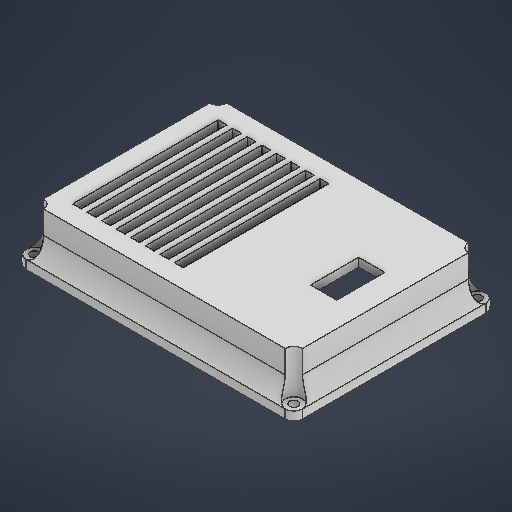
# Autodesk Inventor part: back_cover
Saved by Autodesk Inventor 2026.1 (Build 301233000, 233)
## iProperties
Created: 2026-04-26
Part Number: back_cover
Material: Generic
Document SubType Name: Modeling
Designer: emanuel
Density: 1 g/cm^3
Appearance: Default
Author: emanuel
Autodesk Inventor part; units mm, degrees
ref_plane "YZ Plane" through (0, 0, 0) normal (1, 0, 0) x (0, 1, 0)
ref_plane "XZ Plane" through (0, 0, 0) normal (0, 1, 0) x (-1, 0, 0)
ref_plane "XY Plane" through (0, 0, 0) normal (0, 0, 1) x (1, 0, 0)
sketch "Sketch1" plane through (0, 0, 0) normal (0, 1, 0) x (-1, 0, 0)
  circle A0 centre (44.5, 31.5) radius 1.5
  circle A1 centre (44.5, -31.5) radius 1.5
  circle A2 centre (-44.5, 31.5) radius 1.5
  circle A3 centre (-44.5, -31.5) radius 1.5
  line L0 (44.5, 31.5) -> (44.5, -31.5) construction
  line L1 (41.5, 31.5) -> (41.5, -31.5)
  line L2 (47.5, -31.5) -> (47.5, 31.5)
  arc A4 (47.5, 31.5) -> (41.5, 31.5) centre (44.5, 31.5) ccw
  arc A5 (41.5, -31.5) -> (47.5, -31.5) centre (44.5, -31.5) ccw
  line L3 (44.5, -31.5) -> (-44.5, -31.5) construction
  line L4 (44.5, -28.5) -> (-44.5, -28.5)
  line L5 (-44.5, -34.5) -> (44.5, -34.5)
  arc A6 (44.5, -34.5) -> (44.5, -28.5) centre (44.5, -31.5) ccw
  arc A7 (-44.5, -28.5) -> (-44.5, -34.5) centre (-44.5, -31.5) ccw
  line L6 (-44.5, -31.5) -> (-44.5, 31.5) construction
  line L7 (-41.5, -31.5) -> (-41.5, 31.5)
  line L8 (-47.5, 31.5) -> (-47.5, -31.5)
  arc A8 (-47.5, -31.5) -> (-41.5, -31.5) centre (-44.5, -31.5) ccw
  arc A9 (-41.5, 31.5) -> (-47.5, 31.5) centre (-44.5, 31.5) ccw
  line L9 (-44.5, 31.5) -> (44.5, 31.5) construction
  line L10 (-44.5, 28.5) -> (44.5, 28.5)
  line L11 (44.5, 34.5) -> (-44.5, 34.5)
  arc A10 (-44.5, 34.5) -> (-44.5, 28.5) centre (-44.5, 31.5) ccw
  arc A11 (44.5, 28.5) -> (44.5, 34.5) centre (44.5, 31.5) ccw
  point P0 (44.5, 0)
  point P1 (0, -31.5)
  point P2 (-44.5, 0)
  point P3 (0, 31.5)
  point P4 (41.5, -28.5)
  point P5 (-41.5, -28.5)
  point P6 (-41.5, 28.5)
  point P7 (41.5, 28.5)
  dimension "d2" = 3
  dimension "d3" = 3
  dimension "d4" = 3
  dimension "d5" = 3
  dimension "d6" = 6
  dimension "d7" = 6
  dimension "d8" = 6
  dimension "d9" = 6
  constraints: 32 end point, 16 point on circle, 16 tangent, 12 centre point, 4 midpoint, 4 parallel, 3 perpendicular, 1 vertical
  measures "d2" diameter of A0
  measures "d3" diameter of A1
  measures "d4" diameter of A2
  measures "d5" diameter of A3
  measures "d6" diameter of A5
  measures "d7" diameter of A7
  measures "d8" diameter of A9
  measures "d9" diameter of A11
extrude "Extrusion1" add sketch "Sketch1" along normal blind 3 contours A4 A11 L10 L1 | L1 L10 L7 A9 L11 A4 | L10 A11 L2 A6 L4 L1 | L4 A6 A5 L1 | L1 A5 L5 A8 L7 L4 | L10 A10 A9 L7 | L7 L4 A7 L8 A10 L10 | L7 A8 A7 L4
sketch "Sketch3" plane through (0, 3, 0) normal (0, 1, 0) x (1, 0, 0)
  line L0 (-41.5, -28.5) -> (-41.5, 28.5) projected
  line L1 (41.5, 28.5) -> (41.5, -28.5) projected
  line L2 (-41.5, 28.5) -> (41.5, 28.5)
  line L3 (41.5, 28.5) -> (41.5, -28.5)
  line L4 (41.5, -28.5) -> (-41.5, -28.5)
  line L5 (-41.5, -28.5) -> (-41.5, 28.5)
  circle A0 centre (-44.5, 31.5) radius 1.5 projected
  line L6 (-41.5, 28.5) -> (-44.5, 28.5)
  line L7 (-44.5, 28.5) -> (-44.5, 31.5)
  line L8 (-44.5, 31.5) -> (-41.5, 31.5)
  line L9 (-41.5, 31.5) -> (-41.5, 28.5)
  circle A1 centre (44.5, -31.5) radius 1.5 projected
  line L10 (41.5, -28.5) -> (44.5, -28.5)
  line L11 (44.5, -28.5) -> (44.5, -31.5)
  line L12 (44.5, -31.5) -> (41.5, -31.5)
  line L13 (41.5, -31.5) -> (41.5, -28.5)
  line L14 (44.5, -31.5) -> (-44.5, -31.5)
  line L15 (-44.5, -31.5) -> (-44.5, 31.5)
  line L16 (-44.5, 31.5) -> (44.5, 31.5)
  line L17 (44.5, 31.5) -> (44.5, -31.5)
  line L18 (44.5, 34.5) -> (-44.5, 34.5) projected
  circle A2 centre (-44.5, 31.5) radius 3
  circle A3 centre (-44.5, -31.5) radius 1.5 projected
  arc A4 (-47.5, -31.5) -> (-44.5, -34.5) centre (-44.5, -31.5) ccw projected
  circle A5 centre (-44.5, -31.5) radius 3
  arc A6 (44.5, -34.5) -> (47.5, -31.5) centre (44.5, -31.5) ccw projected
  circle A7 centre (44.5, -31.5) radius 3
  circle A8 centre (44.5, 31.5) radius 3
  point P0 (0, 0)
  point P1 (-44.5, -28.5)
  point P2 (-41.5, -31.5)
  point P3 (44.5, 28.5)
  point P4 (41.5, 31.5)
  constraints: 32 end point, 8 parallel, 4 coincident, 4 horizontal, 4 perpendicular, 1 centre point, 9 other
extrude "Extrusion3" add sketch "Sketch3" along normal blind 15 contours L4 L13 L14 A5 L15 L6 L0 | L9 L16 A8 L17 L10 L1 L2 | L6 A2 L9 | L10 A7 L13
fillet "Fillet2" radius 10 4 edges at (0, 3, 31.5) (44.5, 3, 0) (0, 3, -31.5) (-44.5, 3, 0)
sketch "Sketch4" plane through (0, 18, 0) normal (0, 1, 0) x (1, 0, 0)
  line L0 (41.5, 28.5) -> (41.5, -28.5) projected
  line L1 (41.5, 0) -> (31.5, 0)
  line L2 (27, -8.25) -> (36, -8.25)
  line L3 (36, -8.25) -> (36, 8.25)
  line L4 (36, 8.25) -> (27, 8.25)
  line L5 (27, 8.25) -> (27, -8.25)
  line L6 (27, -8.25) -> (36, 8.25) construction
  line L7 (36, -8.25) -> (27, 8.25) construction
  line L8 (-41.5, -28.5) -> (-41.5, 28.5) projected
  line L9 (-41.5, 0) -> (-31.5, 0)
  line L10 (-31.5, 0) -> (-21.5, 0)
  line L11 (-21.5, 0) -> (-11.5, 0)
  line L12 (-11.5, 0) -> (-1.5, 0)
  line L13 (-38, -25) -> (-35, -25)
  line L14 (-35, -25) -> (-35, 25)
  line L15 (-35, 25) -> (-38, 25)
  line L16 (-38, 25) -> (-38, -25)
  line L17 (-38, -25) -> (-35, 25) construction
  line L18 (-35, -25) -> (-38, 25) construction
  line L19 (-33, -25) -> (-30, -25)
  line L20 (-30, -25) -> (-30, 25)
  line L21 (-30, 25) -> (-33, 25)
  line L22 (-33, 25) -> (-33, -25)
  line L23 (-33, -25) -> (-30, 25) construction
  line L24 (-30, -25) -> (-33, 25) construction
  line L25 (-18, -25) -> (-15, -25)
  line L26 (-15, -25) -> (-15, 25)
  line L27 (-15, 25) -> (-18, 25)
  line L28 (-18, 25) -> (-18, -25)
  line L29 (-18, -25) -> (-15, 25) construction
  line L30 (-15, -25) -> (-18, 25) construction
  line L31 (-23, -25) -> (-20, -25)
  line L32 (-20, -25) -> (-20, 25)
  line L33 (-20, 25) -> (-23, 25)
  line L34 (-23, 25) -> (-23, -25)
  line L35 (-23, -25) -> (-20, 25) construction
  line L36 (-20, -25) -> (-23, 25) construction
  line L37 (-28, -25) -> (-25, -25)
  line L38 (-25, -25) -> (-25, 25)
  line L39 (-25, 25) -> (-28, 25)
  line L40 (-28, 25) -> (-28, -25)
  line L41 (-28, -25) -> (-25, 25) construction
  line L42 (-25, -25) -> (-28, 25) construction
  line L43 (-10, -25) -> (-13, -25)
  line L44 (-13, -25) -> (-13, 25)
  line L45 (-13, 25) -> (-10, 25)
  line L46 (-10, 25) -> (-10, -25)
  line L47 (-10, -25) -> (-13, 25) construction
  line L48 (-13, -25) -> (-10, 25) construction
  line L49 (-8, -25) -> (-5, -25)
  line L50 (-5, -25) -> (-5, 25)
  line L51 (-5, 25) -> (-8, 25)
  line L52 (-8, 25) -> (-8, -25)
  line L53 (-8, -25) -> (-5, 25) construction
  line L54 (-5, -25) -> (-8, 25) construction
  line L55 (-3, -25) -> (0, -25)
  line L56 (0, -25) -> (0, 25)
  line L57 (0, 25) -> (-3, 25)
  line L58 (-3, 25) -> (-3, -25)
  line L59 (-3, -25) -> (0, 25) construction
  line L60 (0, -25) -> (-3, 25) construction
  line L61 (-41.5, 28.5) -> (41.5, 28.5)
  line L62 (41.5, 28.5) -> (41.5, -28.5)
  line L63 (41.5, -28.5) -> (-41.5, -28.5)
  line L64 (-41.5, -28.5) -> (-41.5, 28.5)
  point P0 (0, 0)
  point P1 (-36.5, 0)
  point P2 (-16.5, 0)
  point P3 (-26.5, 0)
  point P4 (-6.5, 0)
  dimension "d25" = 10
  dimension "d26" = 9
  dimension "d27" = 16.5
  dimension "d28" = 10
  dimension "d29" = 10
  dimension "d30" = 10
  dimension "d31" = 10
  dimension "d32" = 3
  dimension "d33" = 50
  dimension "d34" = 3
  dimension "d35" = 50
  dimension "d36" = 3
  dimension "d37" = 50
  dimension "d38" = 3
  dimension "d39" = 50
  dimension "d40" = 3
  dimension "d41" = 50
  dimension "d42" = 3
  dimension "d43" = 50
  dimension "d44" = 3
  dimension "d45" = 50
  dimension "d46" = 3
  dimension "d47" = 50
  constraints: 126 end point, 24 midpoint, 20 parallel, 12 horizontal, 10 perpendicular, 3 point on line
  measures "d25" distance of L1.start L1.end
  measures "d26" distance of L4.end L3.end
  measures "d27" distance of L3.end L2.end
  measures "d28" distance of L9.start L9.end
  measures "d29" distance of L9.end L10.end
  measures "d30" distance of L10.end L11.end
  measures "d31" distance of L11.end L12.end
  measures "d32" distance of L15.end L14.end
  measures "d33" distance of L14.end L13.end
  measures "d34" distance of L21.end L20.end
  measures "d35" distance of L20.end L19.end
  measures "d36" distance of L27.end L26.end
  measures "d37" distance of L26.end L25.end
  measures "d38" distance of L33.end L32.end
  measures "d39" distance of L32.end L31.end
  measures "d40" distance of L39.end L38.end
  measures "d41" distance of L38.end L37.end
  measures "d42" distance of L44.end L45.end
  measures "d43" distance of L43.end L44.end
  measures "d44" distance of L51.end L50.end
  measures "d45" distance of L50.end L49.end
  measures "d46" distance of L57.end L56.end
  measures "d47" distance of L56.end L55.end
extrude "Extrusion4" add sketch "Sketch4" against normal blind 3
body "Solid1"
